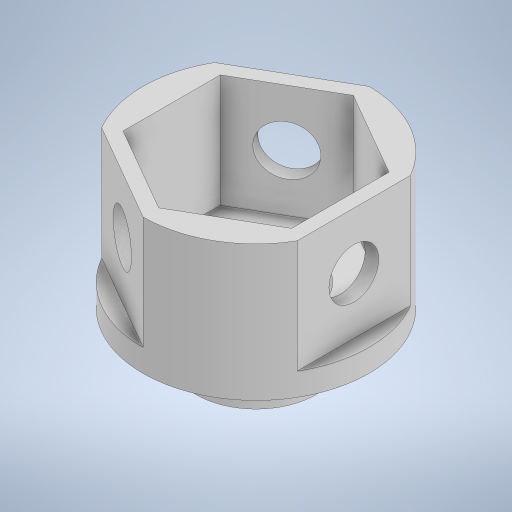
# Autodesk Inventor part: spojkaV2
Saved by Autodesk Inventor 2023 (Build 270158000, 158)
## iProperties
Created: 2023-12-26
Part Number: spojkaV2
Material: Generic
Document SubType Name: Modeling
Designer: alexa
Density: 1 g/cm^3
Appearance: Default
Author: alexa
Autodesk Inventor part; units mm, degrees
ref_plane "YZ Plane" through (0, 0, 0) normal (1, 0, 0) x (0, 1, 0)
ref_plane "XZ Plane" through (0, 0, 0) normal (0, 1, 0) x (-1, 0, 0)
ref_plane "XY Plane" through (0, 0, 0) normal (0, 0, 1) x (1, 0, 0)
sketch "Sketch1" plane through (0, 0, 0) normal (0, 1, 0) x (-1, 0, 0)
  circle A0 centre (0, 0) radius 25
  dimension "d0" = 50
  constraints: 1 centre point, 1 coincident
  measures "d0" diameter of A0
extrude "Extrusion1" add sketch "Sketch1" along normal blind 5
sketch "Sketch2" plane through (0, 5, 0) normal (0, 1, 0) x (1, 0, 0)
  circle A0 centre (0, 0) radius 25
  constraints: 1 centre point, 1 coincident
extrude "Extrusion2" add sketch "Sketch2" along normal blind 25
sketch "Sketch3" plane through (0, 30, 0) normal (0, 1, 0) x (1, 0, 0)
  circle A0 centre (0, 0) radius 25 projected
  line L0 (0, 25) -> (21.6506, 12.5)
  line L1 (21.6506, 12.5) -> (21.6506, -12.5)
  line L2 (21.6506, -12.5) -> (0, -25)
  line L3 (0, -25) -> (-21.6506, -12.5)
  line L4 (-21.6506, -12.5) -> (-21.6506, 12.5)
  line L5 (-21.6506, 12.5) -> (0, 25)
  point P0 (0, -25)
  constraints: 12 end point, 1 coincident, 15 other
extrude "Extrusion3" cut sketch "Sketch3" against normal blind 25 contours A0 L1 | L5 A0 | A0 L3
sketch "Sketch4" plane through (0, 30, 0) normal (0, 1, 0) x (1, 0, 0)
  arc A0 (-21.6506, 12.5) -> (-21.6506, -12.5) centre (0, 0) ccw projected
  line L0 (-21.6506, 12.5) -> (0, 25)
  line L1 (0, 25) -> (21.6506, 12.5)
  line L2 (21.6506, 12.5) -> (21.6506, -12.5)
  line L3 (21.6506, -12.5) -> (0, -25)
  line L4 (0, -25) -> (-21.6506, -12.5)
  line L5 (-21.6506, -12.5) -> (-21.6506, 12.5)
  circle A1 centre (0, 0) radius 25 projected
  line L6 (-18.6506, 10.7679) -> (0, 21.5359)
  line L7 (0, 21.5359) -> (18.6506, 10.7679)
  line L8 (18.6506, 10.7679) -> (18.6506, -10.7679)
  line L9 (18.6506, -10.7679) -> (0, -21.5359)
  line L10 (0, -21.5359) -> (-18.6506, -10.7679)
  line L11 (-18.6506, -10.7679) -> (-18.6506, 10.7679)
  dimension "d7" = 3
  constraints: 24 end point, 2 coincident, 1 parallel, 27 other
  measures "d7" distance between parallel lines of L5 L11
extrude "Extrusion4" cut sketch "Sketch4" against normal blind 25 contours L6 L7 L8 L9 L10 L11
sketch "Sketch5" plane through (0, 5, -25) normal (-0.5, 0, -0.8660254) x (-0.8660254, 0, 0.5)
  circle A0 centre (12.5, 12.5) radius 5.5
  line L0 (0, 0) -> (0, 25) projected
  line L1 (0, 0) -> (25, 0) projected
  line L2 (0, 25) -> (25, 25) projected
  line L3 (25, 25) -> (25, 0) projected
  point P0 (12.5, -5)
  point P1 (25, 12.5)
  dimension "d10" = 11
  dimension "d11" = 12.5
  dimension "d12" = 12.5
  dimension "d13" = 12.5
  dimension "d14" = 12.5
  constraints: 1 centre point, 1 midpoint
  measures "d10" diameter of A0
  measures "d11" distance from line of L0 A0.centre
  measures "d12" distance from line of L1 A0.centre
  measures "d13" distance from line of L2 A0.centre
  measures "d14" distance of point (25, 12.5) A0.centre
extrude "Extrusion5" cut sketch "Sketch5" against normal blind 25 contours A0
pattern_circular "Circular Pattern1" count 3 over 360 about axis through (0, 0, 0) along (0, 1, 0) of "Extrusion5"
sketch "Sketch6" plane through (0, 0, 0) normal (0, -1, 0) x (1, 0, 0)
  circle A0 centre (0, 0) radius 12
  circle A1 centre (0, 0) radius 13.2
  dimension "d20" = 24
  dimension "d21" = 26.4
  constraints: 2 centre point, 2 coincident
  measures "d20" diameter of A0
  measures "d21" diameter of A1
extrude "Extrusion6" add sketch "Sketch6" along normal blind 10
sketch "Sketch7" plane through (0, 0, 0) normal (0, -1, 0) x (1, 0, 0)
  circle A0 centre (0, 0) radius 12 projected
extrude "Extrusion7" cut sketch "Sketch7" against normal blind 10
body "Solid1"
